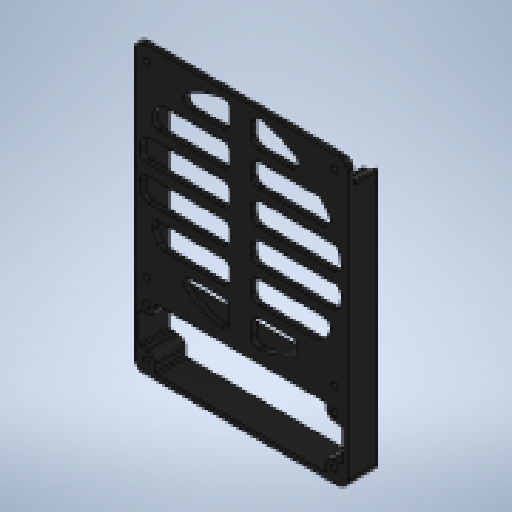
# Autodesk Inventor part: Face Plate
Saved by Autodesk Inventor 2023.2 (Build 272271000, 271)
## iProperties
Created: 2023-08-15
Part Number: Face Plate
Material: UHMW, Black
Document SubType Name: Modeling
Designer: Nathan Cai
Density: 0.94 g/cm^3
Appearance: Smooth - Black
Author: Nathan Cai
Autodesk Inventor part; units mm, degrees
ref_plane "YZ Plane" through (0, 0, 0) normal (1, 0, 0) x (0, 1, 0)
ref_plane "XZ Plane" through (0, 0, 0) normal (0, 1, 0) x (-1, 0, 0)
ref_plane "XY Plane" through (0, 0, 0) normal (0, 0, 1) x (1, 0, 0)
sketch "Sketch1" plane through (0, 0, 0) normal (0, 0, 1) x (1, 0, 0)
  line L0 (-60, -80) -> (60, -80)
  line L1 (60, -80) -> (60, 80)
  line L2 (60, 80) -> (-60, 80)
  line L3 (-60, 80) -> (-60, -80)
  line L4 (-60, -80) -> (60, 80) construction
  line L5 (60, -80) -> (-60, 80) construction
  line L6 (0, 80) -> (0, -80) construction
  line L7 (-52.5, 72.5) -> (52.5, 72.5) construction
  line L8 (52.5, 72.5) -> (52.5, -32.5) construction
  line L9 (52.5, -32.5) -> (-52.5, -32.5) construction
  line L10 (-52.5, -32.5) -> (-52.5, 72.5) construction
  line L11 (-52.5, 72.5) -> (52.5, -32.5) construction
  line L12 (52.5, 72.5) -> (-52.5, -32.5) construction
  circle A0 centre (-52.5, 72.5) radius 2
  circle A1 centre (52.5, 72.5) radius 2
  circle A2 centre (-52.5, -32.5) radius 2
  circle A3 centre (52.5, -32.5) radius 2
  circle A4 centre (-52.5, -72.5) radius 2
  circle A5 centre (52.5, -72.5) radius 2
  circle A6 centre (0, 20) radius 57
  circle A7 centre (52.5, -45.5) radius 2
  circle A8 centre (-52.5, -45.5) radius 2
  point P0 (0, 0)
  point P1 (0, 20)
  dimension "d0" = 120
  dimension "d1" = 160
  dimension "d2" = 105
  dimension "d3" = 105
  dimension "d4" = 7.5
  dimension "d5" = 4
  dimension "d8" = 105
  dimension "d11" = 105
  dimension "d16" = 40
  dimension "d21" = 114
  dimension "d82" = 13
  constraints: 26 end point, 9 centre point, 6 midpoint, 4 parallel, 3 horizontal, 3 vertical, 2 coincident, 2 perpendicular, 1 point on line, 14 other
  measures "d0" distance of L2.end L1.end
  measures "d1" distance of L1.end L0.end
  measures "d2" distance of L8.end L9.end
  measures "d3" distance of L7.end L8.end
  measures "d4" distance between parallel lines of L2 L7
  measures "d5" diameter of A0
  measures "d8" distance of A0.centre A1.centre
  measures "d11" distance of A0.centre A2.centre
  measures "d16" distance of A2.centre A4.centre
  measures "d21" diameter of A6
  measures "d82" distance of A3.centre A7.centre
extrude "Extrusion1" add sketch "Sketch1" along normal blind 3
sketch "Sketch2" plane through (0, 0, 3) normal (0, 0, 1) x (1, 0, 0)
  line L0 (60, -80) -> (60, 80) projected
  line L1 (60, 80) -> (-60, 80) projected
  line L2 (-60, 80) -> (-60, -80) projected
  line L3 (-60, -80) -> (60, -80) projected
  circle A0 centre (-52.5, -72.5) radius 2 projected
  circle A1 centre (52.5, -72.5) radius 2 projected
  circle A2 centre (0, 20) radius 57 projected
  circle A3 centre (52.5, -32.5) radius 2 projected
  circle A4 centre (-52.5, -32.5) radius 2 projected
  circle A5 centre (52.5, 72.5) radius 2 projected
  circle A6 centre (-52.5, 72.5) radius 2 projected
  line L4 (0, 73.4838) -> (0, -23.4838) construction
  line L5 (-6, 77) -> (6, 77) construction
  line L6 (6, 77) -> (6, -37)
  line L7 (6, -37) -> (-6, -37) construction
  line L8 (-6, -37) -> (-6, 77)
  line L9 (-6, 77) -> (6, -37) construction
  line L10 (6, 77) -> (-6, -37) construction
  circle A7 centre (0, 20) radius 57 projected
  line L11 (-44.9889, 61) -> (44.9889, 61)
  line L12 (44.9889, 61) -> (44.9889, 55)
  line L13 (44.9889, 55) -> (-44.9889, 55)
  line L14 (-44.9889, 55) -> (-44.9889, 61)
  line L15 (-44.9889, 61) -> (44.9889, 55) construction
  line L16 (44.9889, 61) -> (-44.9889, 55) construction
  line L17 (-57, 17) -> (57, 17)
  line L18 (57, 17) -> (57, 23)
  line L19 (57, 23) -> (-57, 23)
  line L20 (-57, 23) -> (-57, 17)
  line L21 (-57, 17) -> (57, 23) construction
  line L22 (57, 17) -> (-57, 23) construction
  line L23 (-54.7083, 42) -> (54.7083, 42)
  line L24 (54.7083, 42) -> (54.7083, 36)
  line L25 (54.7083, 36) -> (-54.7083, 36)
  line L26 (-54.7083, 36) -> (-54.7083, 42)
  line L27 (-54.7083, 42) -> (54.7083, 36) construction
  line L28 (54.7083, 42) -> (-54.7083, 36) construction
  line L29 (-57, 20) -> (57, 20) construction
  line L30 (-44.9889, -21) -> (44.9889, -21)
  line L31 (44.9889, -21) -> (44.9889, -15)
  line L32 (44.9889, -15) -> (-44.9889, -15)
  line L33 (-44.9889, -15) -> (-44.9889, -21)
  line L34 (-44.9889, -21) -> (44.9889, -15) construction
  line L35 (44.9889, -21) -> (-44.9889, -15) construction
  line L36 (-54.7083, -2) -> (54.7083, -2)
  line L37 (54.7083, -2) -> (54.7083, 4)
  line L38 (54.7083, 4) -> (-54.7083, 4)
  line L39 (-54.7083, 4) -> (-54.7083, -2)
  line L40 (-54.7083, -2) -> (54.7083, 4) construction
  line L41 (54.7083, -2) -> (-54.7083, 4) construction
  point P0 (0, 58)
  point P1 (0, 39)
  point P2 (0, -18)
  point P3 (0, 1)
  point P4 (6, 61)
  point P5 (6, 76.6833)
  point P6 (-6, 76.6833)
  point P7 (-6, 61)
  point P8 (-39.598, 61)
  point P9 (-44.9889, 55)
  point P10 (-6, 55)
  point P11 (-6, 42)
  point P12 (-52.5833, 42)
  point P13 (-6, 36)
  point P14 (-6, 23)
  point P15 (-56.921, 23)
  point P16 (-56.921, 17)
  point P17 (-6, 17)
  point P18 (-6, 4)
  point P19 (-54.7083, 4)
  point P20 (-52.5833, -2)
  point P21 (-6, -2)
  point P22 (-6, -15)
  point P23 (-44.9889, -15)
  point P24 (-39.598, -21)
  point P25 (-6, -21)
  point P26 (-6, -36.6833)
  point P27 (6, -36.6833)
  point P28 (6, -21)
  point P29 (39.598, -21)
  point P30 (44.9889, -15)
  point P31 (6, -15)
  point P32 (6, -2)
  point P33 (52.5833, -2)
  point P34 (54.7083, 4)
  point P35 (6, 4)
  point P36 (6, 17)
  point P37 (56.921, 17)
  point P38 (56.921, 23)
  point P39 (6, 23)
  point P40 (6, 36)
  point P41 (54.7083, 36)
  point P42 (52.5833, 42)
  point P43 (6, 42)
  point P44 (6, 55)
  point P45 (44.9889, 55)
  point P46 (39.598, 61)
  dimension "d106" = 12
  dimension "d108" = 6
  dimension "d110" = 35
  dimension "d111" = 6
  dimension "d112" = 6
  dimension "d113" = 13
  constraints: 76 end point, 10 midpoint, 10 symmetric about line, 8 parallel, 6 horizontal, 4 perpendicular, 4 point on line, 2 vertical, 4 other
  measures "d106" distance of L6.end L7.end
  measures "d108" distance of L11.end L12.end
  measures "d110" distance from line of point (0, 20) L13
  measures "d111" distance between parallel lines of L19 L17
  measures "d112" distance between parallel lines of L25 L23
  measures "d113" distance between parallel lines of L19 L25
extrude "Extrusion2" add sketch "Sketch2" against normal up to surface (3 mm away) contours A2 L17 L6 L19 | L25 L6 L23 A2 | L19 L8 L25 L6 | L6 L17 L8 L19 | A2 L36 L6 L38 | L6 L38 L8 L17 | L25 L8 L23 L6 | L8 L17 A2 L19 | L6 L36 L8 L38 | L13 L6 L11 A2 | L23 L8 L13 L6 | L25 A2 L23 L8 | A2 L30 L6 L32 | L6 L32 L8 L36 | L8 L36 A2 L38 | L13 L8 L11 L6 | L6 L30 L8 L32 | L6 L11 L8 A2 | L13 A2 L11 L8 | A2 L8 L30 L6 | L8 L30 A2 L32
fillet "Fillet4" radius 4 44 edges at (44.9889, -15, 1.5) (39.598, -21, 1.5) (6, -36.6833, 1.5) (6, -21, 1.5) (6, -15, 1.5) (-6, -15, 1.5) (-6, -36.6833, 1.5) (-6, -21, 1.5) (-39.598, -21, 1.5) (-44.9889, -15, 1.5) (-52.5833, -2, 1.5) (-6, -2, 1.5) (6, -2, 1.5) (52.5833, -2, 1.5) (54.7083, 4, 1.5) (6, 4, 1.5) (-6, 4, 1.5) (-54.7083, 4, 1.5) (-56.921, 17, 1.5) (-56.921, 23, 1.5) (-6, 23, 1.5) (-6, 17, 1.5) (6, 17, 1.5) (6, 23, 1.5) (56.921, 23, 1.5) (56.921, 17, 1.5) (54.7083, 36, 1.5) (6, 36, 1.5) (-6, 36, 1.5) (-54.7083, 36, 1.5) (-52.5833, 42, 1.5) (-6, 42, 1.5) (-6, 55, 1.5) (-44.9889, 55, 1.5) (-39.598, 61, 1.5) (-6, 61, 1.5) (-6, 76.6833, 1.5) (6, 76.6833, 1.5) (6, 61, 1.5) (39.598, 61, 1.5) (44.9889, 55, 1.5) (52.5833, 42, 1.5) (6, 55, 1.5) (6, 42, 1.5)
sketch "Sketch3" plane through (0, 0, 0) normal (0, 0, -1) x (-1, 0, 0)
  line L0 (-60, -80) -> (-60, 80) projected
  line L1 (-60, -80) -> (60, -80)
  line L2 (60, -80) -> (60, -40)
  line L3 (60, -40) -> (-60, -40)
  line L4 (-60, -40) -> (-60, -80)
  line L5 (-57, -43) -> (57, -43)
  line L6 (57, -43) -> (57, -77)
  line L7 (57, -77) -> (-57, -77)
  line L8 (-57, -77) -> (-57, -43)
  circle A0 centre (-52.5, -72.5) radius 2 projected
  circle A1 centre (-52.5, -72.5) radius 4.5
  line L9 (-48, -72.5) -> (-48, -77)
  line L10 (-52.5, -68) -> (-57, -68)
  line L11 (0, -77) -> (0, -43) construction
  circle A2 centre (52.5, -72.5) radius 2
  circle A3 centre (52.5, -72.5) radius 4.5
  line L12 (48, -72.5) -> (48, -77)
  line L13 (52.5, -68) -> (57, -68)
  line L14 (-60, 80) -> (60, 80) projected
  circle A4 centre (-52.5, -45.5) radius 2 projected
  arc A5 (-52.5, -50) -> (-48, -45.5) centre (-52.5, -45.5) ccw
  line L15 (-52.5, -50) -> (-57, -50)
  line L16 (-48, -45.5) -> (-48, -43)
  arc A6 (48, -45.5) -> (52.5, -50) centre (52.5, -45.5) ccw
  line L17 (52.5, -50) -> (57, -50)
  line L18 (48, -45.5) -> (48, -43)
  circle A7 centre (52.5, -45.5) radius 2 projected
  line L19 (-60, 80) -> (60, 80) projected
  line L20 (-60, 80) -> (60, 80)
  line L21 (60, 80) -> (60, -40)
  line L22 (60, -40) -> (-60, -40)
  line L23 (-60, -40) -> (-60, 80)
  line L24 (57, 77) -> (-57, 77)
  line L25 (-57, 77) -> (-57, -40)
  line L26 (57, -40) -> (57, 77)
  circle A8 centre (-52.5, 72.5) radius 2 projected
  circle A9 centre (-52.5, 72.5) radius 4.5
  circle A10 centre (-52.5, 72.5) radius 7.5
  line L27 (60, 80) -> (-60, 80)
  line L28 (-60, 80) -> (-60, 65)
  line L29 (-60, 65) -> (60, 65)
  line L30 (60, 65) -> (60, 80)
  circle A11 centre (-55, 61) radius 2
  circle A12 centre (-55, 61) radius 4
  line L31 (-55, 57) -> (-57, 57)
  line L32 (-51, 61) -> (-51, 65)
  line L33 (0, 0) -> (0, -40)
  circle A13 centre (55, 61) radius 2
  circle A14 centre (55, 61) radius 4
  line L34 (55, 57) -> (57, 57)
  line L35 (51, 61) -> (51, 65)
  point P0 (60, 65)
  point P1 (57, 65)
  point P2 (-57, 66.5)
  point P3 (-60, 72.5)
  point P4 (57, 61)
  point P5 (-52.5, 65)
  point P6 (-57, 61)
  dimension "d74" = 120
  dimension "d75" = 40
  dimension "d76" = 3
  dimension "d77" = 160
  dimension "d115" = 3
  dimension "d116" = 3
  dimension "d117" = 3
  dimension "d118" = 4
  dimension "d119" = 8
  constraints: 66 end point, 17 symmetric about line, 13 tangent, 12 point on circle, 11 centre point, 11 perpendicular, 9 parallel, 9 point on line, 7 coincident, 3 horizontal, 3 midpoint, 8 other
  measures "d74" distance of L3.end L2.end
  measures "d75" distance of L2.end L1.end
  measures "d76" distance between parallel lines of L0 L8
  measures "d77" distance between parallel lines of L14 L1
  measures "d115" distance between parallel lines of L20 L24
  measures "d116" distance between parallel lines of L0 L25
  measures "d117" distance between parallel lines of L21 L26
  measures "d118" diameter of A11
  measures "d119" diameter of A12
extrude "Extrusion3" add sketch "Sketch3" along normal blind 14 contours L0 L3 L2 L1 | L0 L29 L25 A12 L3 | L0 A10 L25 L29 | L3 L26 A14 L29 L21 | L29 A12 L25 | L25 A10 L29 | L25 A12 L31 | A12 L25 | L25 A12 | L29 L32 A12 | L34 A14 L26 | L26 A14 L29 | A14 L26 | L26 A14 | A14 L35 L29 | L5 L16 A5 L15 L8 | L5 L6 L17 A6 L18 | L10 A1 L8 | A1 L7 L8 | A1 | A1 L9 L7 | L6 A3 L13 | A3 | L6 L7 A3 | L12 A3 L7
extrude "Extrusion6" cut sketch "Sketch3" against normal blind 10 contours L5 L18 A6 L17 L6 L13 A3 L12 L7 L9 A1 L10 L8 L15 A5 L16
fillet "Fillet1" radius 5 4 edges at (60, 80, 1.5) (60, -80, -5.5) (-60, -80, -5.5) (-60, 80, 1.5)
fillet "Fillet3" radius 1 24 edges at (48, -43, 1.5) (48, -43, -7) (57, -50, 1.5) (57, -50, -7) (57, -68, 1.5) (57, -68, -7) (48, -77, 1.5) (48, -77, -7) (-48, -77, 1.5) (-48, -77, -7) (-57, -68, 1.5) (-57, -68, -7) (-57, -50, 1.5) (-57, -50, -7) (-48, -43, 1.5) (-48, -43, -7) (57, -40, -7) (-57, -40, -7) (60, 72.5, -7) (51, 65, -7) (57, 57, -7) (-60, 65, -7) (-51, 65, -7) (-57, 57, -7)
equation "\"d8\" = d3"
equation "\"d11\" = d2"
equation "\"d111\" = d108"
equation "\"d112\" = d108"
body "Solid1"
